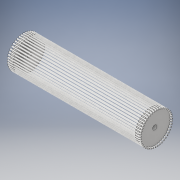
# Autodesk Inventor part: roller
Saved by Autodesk Inventor 2019 (Build 230136000, 136)
## iProperties
Created: 2019-04-01
Part Number: roller
Material: Generic
Document SubType Name: Modeling
Designer: Tesler
Density: 1 g/cm^3
Appearance: Default
Author: Tesler
Autodesk Inventor part; units mm, degrees
ref_plane "YZ Plane" through (0, 0, 0) normal (1, 0, 0) x (0, 1, 0)
ref_plane "XZ Plane" through (0, 0, 0) normal (0, 1, 0) x (-1, 0, 0)
sketch "Sketch1" plane through (0, 0, 0) normal (1, 0, 0) x (0, 1, 0)
  circle A0 centre (0, 0) radius 20
  dimension "d0" = 40
  constraints: 1 centre point, 1 coincident
  measures "d0" diameter of A0
extrude "Extrusion1" add sketch "Sketch1" along normal blind 5
ref_plane "Work Plane1" through (160, 0, 0) normal (1, 0, 0) x (0, 0, -1)
sketch "Sketch2" plane through (160, 0, 0) normal (1, 0, 0) x (0, 0, -1)
  circle A0 centre (0, 0) radius 20 projected
  circle A1 centre (0, 0) radius 20
  constraints: 1 centre point, 1 coincident, 1 concentric
extrude "Extrusion2" add sketch "Sketch2" along normal blind 5
sketch "Sketch3" plane through (165, 0, 0) normal (1, 0, 0) x (0, 0, -1)
  circle A0 centre (0, 0) radius 2.75
  dimension "d6" = 5.5
  constraints: 1 centre point, 1 coincident
  measures "d6" diameter of A0
extrude "Extrusion3" cut sketch "Sketch3" against normal blind 200
sketch "Sketch4" plane through (165, 0, 0) normal (1, 0, 0) x (0, 0, -1)
  circle A0 centre (0, 0) radius 20 projected
  circle A1 centre (0, 20) radius 0.75
  circle A2 centre (0, 0) radius 20 projected
  dimension "d9" = 1.5
  constraints: 1 centre point, 1 vertical alignment, 2 other
  measures "d9" diameter of A1
extrude "Extrusion4" add sketch "Sketch4" against normal blind 167.5 and the other way blind 2.5 contours A1 A0 | A0 A1 picked at (0.0298, 19.7507) picked at (0.028, 20.2474)
pattern_circular "Circular Pattern1" count 45 over 360 about axis through (0, 0, 0) along (1, 0, 0) of "Extrusion4"
body "Solid1"
